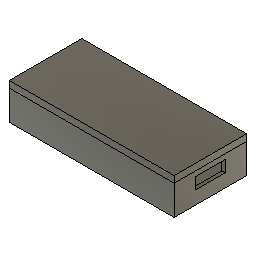
grubswitch (Autodesk Fusion 360 design; units mm, degrees)
Autodesk Fusion 360 part; units mm, degrees
sketch "Sketch1" plane through (0, 0, 0) normal (0, 0, 1) x (1, 0, 0)
  line L0 (-25, 11) -> (25, 11)
  line L1 (25, 11) -> (25, -11)
  line L2 (25, -11) -> (-25, -11)
  line L3 (-25, -11) -> (-25, 11)
  line L4 (-25, 11) -> (25, -11) construction
  line L5 (25, 11) -> (-25, -11) construction
  line L6 (-17, 6.5) -> (-7, 6.5)
  line L7 (-7, 6.5) -> (-7, -6.5)
  line L8 (-7, -6.5) -> (-17, -6.5)
  line L9 (-17, -6.5) -> (-17, 6.5)
  line L10 (0, 0) -> (-25, 0) construction
  line L11 (-17, 6.5) -> (-17, 9.5)
  line L12 (-17, 9.5) -> (24, 9.5)
  line L13 (24, 9.5) -> (24, 0)
  line L14 (-17, -6.5) -> (-17, -9.5)
  line L15 (-17, -9.5) -> (24, -9.5)
  line L16 (24, -9.5) -> (24, 0)
  point P0 (-17, 0)
  dimension "d1" = 50
  dimension "d2" = 22
  dimension "d3" = 10
  dimension "d4" = 13
  dimension "d5" = 8
  dimension "d6" = 1.5
  dimension "d7" = 1
  constraint horizontal L0
  constraint perpendicular L0 L1
  constraint parallel L0 L2
  constraint parallel L1 L3
  constraint coincident L4 L10.start
  constraint coincident L5 L10.start
  constraint coincident L10.start origin
  constraint horizontal L6
  constraint vertical L7
  constraint horizontal L8
  constraint vertical L9
  constraint midpoint L9 P0
  constraint midpoint L3 L10.end
  constraint coincident P0 L10
  constraint perpendicular L6 L11
  constraint perpendicular L11 L12
  constraint perpendicular L12 L13
  constraint symmetric L6.start L10 L8.end
  constraint symmetric L10 L11.end L14.end
  constraint symmetric L10 L12.end L15.end
  constraint symmetric L10 L13.end L16.end
  constraint coincident L13.end L16.end
  measures "d1" distance of L1.end L2.end
  measures "d2" distance of L0.end L1.end
  measures "d3" distance of L6.start L6.end
  measures "d4" distance of L6.start L8.end
  measures "d5" distance of L3 L9
  measures "d6" distance of L0 L12
  measures "d7" distance of L1 L13
extrude "Extrude1" add sketch "Sketch1" along normal blind 1 contours L6 L7 L8 L9 makes body 1
extrude "Extrude2" add sketch "Sketch1" along normal blind 2 contours L6 L7 L8 L11 L12 L13 L14 L15 L16 bodies 1
extrude "Extrude3" add sketch "Sketch1" along normal blind 9 bodies 1
sketch "Sketch2" plane through (-25, 0, 0) normal (-1, 0, 0) x (0, -1, 0)
  line L0 (-11, 0) -> (11, 0)
  line L1 (11, 0) -> (11, 9)
  line L2 (11, 9) -> (-11, 9)
  line L3 (-11, 9) -> (-11, 0)
  line L4 (0, 0) -> (0, 9) construction
  circle A0 centre (0, 5) radius 3
  dimension "d15" = 6
  dimension "d16" = 4
  constraint coincident L4.start origin
  constraint midpoint L2 L4.end
  constraint coincident L4 A0.centre
  measures "d15" diameter of A0
  measures "d16" distance of L2 A0.centre
extrude "Extrude4" cut sketch "Sketch2" against normal blind 10 contours A0 bodies 1
chamfer "Chamfer1" distance 3 distance2 1 1 edges at (-7, 0, 2) measured on face at (13.6667, 2.1667, 2) on bodies 1
chamfer "Chamfer2" distance 0.3 angle 45 2 edges at (-10.5, 6.5, 2) (-10.5, -6.5, 2) on bodies 1
sketch "Sketch3" plane through (24, 0, 0) normal (-1, 0, 0) x (0, -1, 0)
  line L0 (-9.5, 2) -> (9.5, 2)
  line L1 (9.5, 2) -> (9.5, 9)
  line L2 (9.5, 9) -> (-9.5, 9)
  line L3 (-9.5, 9) -> (-9.5, 2)
  line L4 (-4.5, 7.5) -> (4.5, 7.5)
  line L5 (4.5, 7.5) -> (4.5, 4)
  line L6 (4.5, 4) -> (-4.5, 4)
  line L7 (-4.5, 4) -> (-4.5, 7.5)
  line L8 (0, 9) -> (0, 2) construction
  point P0 (0, 7.5)
  dimension "d22" = 9
  dimension "d23" = 3.5
  dimension "d24" = 2
  constraint horizontal L4
  constraint vertical L5
  constraint horizontal L6
  constraint vertical L7
  constraint midpoint L2 L8.start
  constraint midpoint L0 L8.end
  constraint midpoint L4 P0
  constraint coincident L8 P0
  measures "d22" distance of L4.start L4.end
  measures "d23" distance of L4.start L6.end
  measures "d24" distance of L0 L6
extrude "Extrude5" cut sketch "Sketch3" against normal blind 2 contours L4 L5 L6 L7 bodies 1
sketch "Sketch4" plane through (0, 0, 9) normal (0, 0, 1) x (-1, 0, 0)
  line L0 (17, 9.5) -> (17, -9.5)
  line L1 (17, -9.5) -> (-24, -9.5)
  line L2 (-24, -9.5) -> (-24, 9.5)
  line L3 (-24, 9.5) -> (17, 9.5)
  line L4 (25, 11) -> (-25, 11)
  line L5 (-25, 11) -> (-25, -11)
  line L6 (-25, -11) -> (25, -11)
  line L7 (25, -11) -> (25, 11)
  line L8 (5, 9.5) -> (5, -9.5)
  dimension "d31" = 12
  constraint coincident L3 L8.start
  constraint coincident L1 L8.end
  constraint perpendicular L1 L8
  measures "d31" distance of L0 L8
extrude "Extrude6" add sketch "Sketch4" along normal blind 2 separate body contours L0 L1 L3 L8 | L1 L2 L3 L8 | L4 L5 L6 L7 makes body 2
extrude "Extrude7" add sketch "Sketch4" against normal blind 1.5 contours L1 L2 L3 L8 bodies 2
sketch "Sketch5" plane through (0, 9.5, 0) normal (0, -1, 0) x (1, 0, 0)
  line L0 (-17, 2) -> (24, 2)
  line L1 (24, 2) -> (24, 9)
  line L2 (24, 9) -> (-17, 9)
  line L3 (-17, 9) -> (-17, 2)
  line L4 (-17, 7.5) -> (24, 7.5)
  dimension "d32" = 1.5
  constraint coincident L3 L4.start
  constraint coincident L1 L4.end
  constraint perpendicular L1 L4
  measures "d32" distance of L2 L4
extrude "Extrude8" add sketch "Sketch5" along normal blind 1 draft -45 contours L1 L2 L3 L4 bodies 1
mirror "Mirror1" about plane through (0, 0, 0) normal (0, 1, 0) of "Extrude8"
extrude "Extrude9" cut 1 faces at (4.6667, 9.5, 8.5) along direction (0, -1, 0) blind 1 draft -45 on bodies 2 bodies 2
extrude "Extrude10" cut 1 faces at (14.3333, -9.5, 8.5) along direction (0, 1, 0) blind 1 draft -45 on bodies 2 bodies 2
named bodies: "grubswitch_body", "grubswitch_lid"
